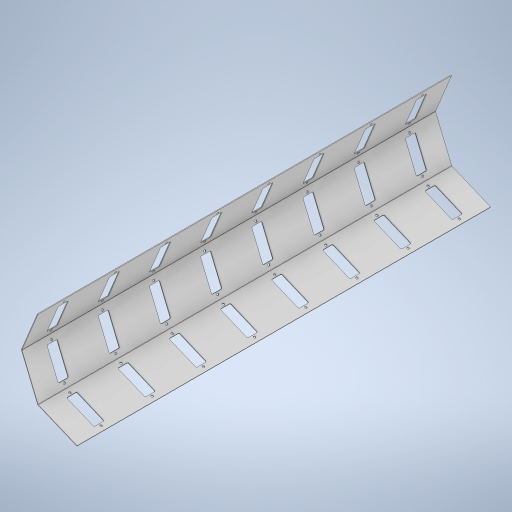
# Autodesk Inventor part: ДМС 100 Барабан Лист №1
Saved by Autodesk Inventor 2024.2 (Build 282272000, 272)
## iProperties
Created: 2024-04-28
Part Number: ДМС 100 Барабан Лист №1
Material: Generic
Document SubType Name: Sheet Metal
Designer: pokla
Density: 1 g/cm^3
Appearance: Default
Sheet Metal Rule: Default
Author: pokla
Autodesk Inventor part; units mm, degrees
ref_plane "YZ Plane" through (0, 0, 0) normal (1, 0, 0) x (0, 1, 0)
ref_plane "XZ Plane" through (0, 0, 0) normal (0, 1, 0) x (-1, 0, 0)
ref_plane "XY Plane" through (0, 0, 0) normal (0, 0, 1) x (1, 0, 0)
sketch "Sketch2" plane through (0, 0, 0) normal (0, 0, 1) x (1, 0, 0)
  line L0 (0, 273.8452) -> (193.6378, 193.6378) construction
  line L1 (193.6378, 193.6378) -> (273.8452, 0) construction
  line L2 (273.8452, 0) -> (193.6378, -193.6378) construction
  line L3 (193.6378, -193.6378) -> (0, -273.8452) construction
  line L4 (0, -273.8452) -> (-193.6378, -193.6378) construction
  line L5 (-193.6378, -193.6378) -> (-273.8452, 0) construction
  line L6 (-273.8452, 0) -> (-193.6378, 193.6378) construction
  line L7 (-193.6378, 193.6378) -> (0, 273.8452) construction
  line L8 (-272.8942, -2.2961) -> (-194.5889, -191.3417)
  line L9 (-191.3417, -194.5889) -> (-2.3097, -272.8885)
  arc A0 (-272.8942, 2.2961) -> (-272.8942, -2.2961) centre (-267.3509, 0) ccw
  arc A1 (-194.5889, -191.3417) -> (-191.3417, -194.5889) centre (-189.0456, -189.0456) ccw
  line L10 (-272.8942, 2.2961) -> (-194.5945, 191.3281)
  point P0 (0, 0)
  point P1 (0, 0)
  dimension "d58" = 6
  dimension "d59" = 6
  dimension "d70" = 2.5
  dimension "d72" = 2.5
  dimension "d74" = 506
  measures "d58" radius of A0
  measures "d59" radius of A1
  measures "d70" distance of L3.end L9.end
  measures "d72" distance of L6.end L10.end
  measures "d74" distance between parallel lines of L1 L8
contour flange "Contour Flange3" sketch "Sketch2" thickness 3 bend radius 3 width 2020 along (0, 0, -1) mid plane no both sides no wall seen from (-96.8257, -233.7387, 0) lies toward (0.3826834, 0.9238795, 0) curves L9 A1 L8 A0 L10
bend "Bend6"
corner "Corner6"
sketch "Sketch11" plane through (-270.1225, -1.1481, 0) normal (0.9238795, 0.3826834, 0) x (0, 0, -1)
  line L0 (0, 0) -> (2020, 0) projected
  line L1 (0, -204.6215) -> (0, 0) projected
  line L2 (0, -204.6215) -> (2020, -204.6215) projected
  line L3 (2020, -204.6215) -> (2020, 0) projected
  circle A0 centre (885, -19.8107) radius 5
  circle A1 centre (885, -184.8107) radius 5
  line L4 (860, -29.8107) -> (910, -29.8107)
  line L5 (910, -29.8107) -> (910, -174.8107)
  line L6 (910, -174.8107) -> (860, -174.8107)
  line L7 (860, -174.8107) -> (860, -29.8107)
  line L8 (860, -102.3107) -> (910, -102.3107) construction
  point P0 (0, -102.3107)
  point P1 (2020, -102.3107)
  point P2 (885, -29.8107)
  point P3 (885, -174.8107)
  point P4 (1010, 0)
  dimension "d141" = 50
  dimension "d142" = 145
  dimension "d143" = 10
  dimension "d145" = 125
  dimension "d146" = 10
  constraints: 10 end point, 6 midpoint, 2 centre point, 2 horizontal, 2 parallel, 2 vertical alignment, 1 equal radius, 1 horizontal alignment, 1 perpendicular, 1 other
  measures "d141" distance of L4.start L4.end
  measures "d142" distance of L4.end L5.end
  measures "d143" distance from line of A0.centre L4
  measures "d145" horizontal distance of A0.centre point (1010, 0)
  measures "d146" diameter of A0
extrude "Extrusion4" cut sketch "Sketch11" against normal blind 10 contours A0 | A1 | L4 L5 L6 L7
fillet "Fillet1" radius 5 4 edges at (-260.1003, -29.2636, -910) (-260.1003, -29.2636, -860) (-204.6112, -163.2261, -860) (-204.6112, -163.2261, -910)
pattern_circular "Circular Pattern2" count 3 over 90 about axis through (0, 0, -10) along (0, 0, 1) of "Extrusion4", "Fillet1" both ways yes
pattern_linear "Rectangular Pattern2" count 8 spacing 250 along (0, 0, -1) of "Extrusion4", "Fillet1", "Circular Pattern2" first direction both ways yes
equation "\"d58\" = BendRadius + Thickness"
equation "\"d59\" = BendRadius + Thickness"
equation "\"d74\" = Барабан_габарит_по_кассетам"
equation "\"d75\" = Thickness"
equation "\"d76\" = BendReliefWidth"
equation "\"d77\" = BendReliefDepth"
equation "\"d78\" = MinimumRemnant"
equation "\"d79\" = TransitionRadius"
equation "\"d80\" = Барабан_длина_листа"
equation "\"d81\" = BendRadius"
equation "\"d83\" = CornerReliefSize"
equation "\"d84\" = GapSize"
equation "\"d85\" = JacobiRadiusSize"
equation "\"BendRadius\" = Thickness"
equation "\"BendReliefWidth\" = Thickness"
equation "\"BendReliefDepth\" = 0.5 * Thickness"
equation "\"CornerReliefSize\" = 4 * Thickness"
equation "\"MinimumRemnant\" = 2 * Thickness"
equation "\"TransitionRadius\" = BendRadius"
equation "\"JacobiRadiusSize\" = BendRadius"
equation "\"GapSize\" = Thickness"
equation "\"Thickness\" = 3"
equation "\"Барабан_габарит_по_кассетам\" = 506"
equation "\"Барабан_длина_листа\" = 2020"
body "Solid3"
